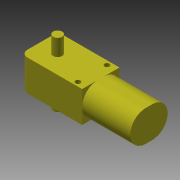
# Autodesk Inventor part: Motor_gerade
Saved by Autodesk Inventor 2015 (Build 190159000, 159)
## iProperties
Created: 2015-03-02
Part Number: Motor_gerade
Material: Generisch
Document SubType Name: Modeling
Designer: TowerSebi
Density: 1 g/cm^3
Appearance: Kanariengelb
Author: TowerSebi
Autodesk Inventor part; units mm, degrees
ref_plane "YZ Plane" through (0, 0, 0) normal (1, 0, 0) x (0, 1, 0)
ref_plane "XZ Plane" through (0, 0, 0) normal (0, 1, 0) x (-1, 0, 0)
ref_plane "XY Plane" through (0, 0, 0) normal (0, 0, 1) x (1, 0, 0)
sketch "Skizze1" plane through (0, 0, 0) normal (0, 0, 1) x (1, 0, 0)
  line L0 (0, 0) -> (37, 0)
  line L1 (37, 0) -> (37, 22.5)
  line L2 (37, 22.5) -> (0, 22.5)
  line L3 (0, 22.5) -> (0, 0)
  dimension "d0" = 37
  dimension "d1" = 22.5
  constraints: 8 end point, 2 parallel, 1 horizontal, 1 perpendicular
  measures "d0" distance of L1.end L2.end
  measures "d1" distance of L2.end L0.start
extrude "Extrusion1" add sketch "Skizze1" along normal blind 18.7
sketch "Skizze2" plane through (37, 0, 0) normal (1, 0, 0) x (0, 0, -1)
  line L0 (0, 0) -> (0, 22.5) projected
  line L1 (-9.35, 13.157) -> (-9.35, 9.3514) construction
  line L2 (-18.7, 13.157) -> (-18.7, 9.3514)
  line L3 (0, 9.3514) -> (0, 13.157)
  arc A0 (0, 13.157) -> (-18.7, 13.157) centre (-9.35, 13.157) ccw
  arc A1 (-18.7, 9.3514) -> (0, 9.3514) centre (-9.35, 9.3514) ccw
  point P0 (-9.35, 11.2542)
  constraints: 8 end point, 4 point on circle, 4 tangent, 2 centre point, 2 parallel, 1 midpoint
extrude "Extrusion2" add sketch "Skizze2" along normal blind 29
sketch "Skizze3" plane through (0, 0, 18.7) normal (0, 0, 1) x (1, 0, 0)
  line L0 (37, 22.5) -> (0, 22.5) projected
  line L1 (0, 22.5) -> (0, 0) projected
  circle A0 centre (11, 11.25) radius 2.75
  dimension "d6" = 11
  dimension "d7" = 11.25
  dimension "d21" = 5.5
  constraints: 1 centre point
  measures "d6" distance from line of L1 A0.centre
  measures "d7" distance from line of L0 A0.centre
  measures "d21" diameter of A0
extrude "Extrusion3" add sketch "Skizze3" along normal blind 10
sketch "Skizze4" plane through (0, 0, 0) normal (0, 0, -1) x (-1, 0, 0)
  line L0 (0, 0) -> (-37, 0) projected
  line L1 (0, 22.5) -> (0, 0) projected
  circle A0 centre (-11, 11.25) radius 2.75
  dimension "d10" = 5.5
  dimension "d11" = 11
  dimension "d12" = 11.25
  constraints: 1 centre point
  measures "d10" diameter of A0
  measures "d11" distance from line of L1 A0.centre
  measures "d12" distance from line of L0 A0.centre
extrude "Extrusion4" add sketch "Skizze4" along normal blind 10
sketch "Skizze5" plane through (0, 0, 0) normal (0, 0, -1) x (-1, 0, 0)
  line L0 (0, 0) -> (-37, 0) projected
  line L1 (0, 22.5) -> (0, 0) projected
  line L2 (-37, 22.5) -> (0, 22.5) projected
  circle A0 centre (-22.5, 11.25) radius 2
  dimension "d15" = 4
  dimension "d16" = 11.25
  dimension "d17" = 22.5
  dimension "d18" = 11.25
  constraints: 1 centre point
  measures "d15" diameter of A0
  measures "d16" distance from line of L0 A0.centre
  measures "d17" distance from line of L1 A0.centre
  measures "d18" distance from line of L2 A0.centre
extrude "Extrusion5" add sketch "Skizze5" along normal blind 2
sketch "Skizze6" plane through (0, 0, 0) normal (-1, 0, 0) x (0, 0, 1)
  line L0 (0, 22.5) -> (0, 0) projected
  line L1 (18.7, 22.5) -> (18.7, 0) projected
  line L2 (7.85, 13.5868) -> (10.85, 13.5868)
  line L3 (10.85, 13.5868) -> (10.85, 8.5868)
  line L4 (10.85, 8.5868) -> (7.85, 8.5868)
  line L5 (7.85, 8.5868) -> (7.85, 13.5868)
  line L6 (9.35, 13.5868) -> (9.35, 8.5868)
  dimension "d22" = 3
  dimension "d23" = 5
  dimension "d25" = 18.7
  dimension "d26" = 7.85
  dimension "d27" = 7.85
  constraints: 10 end point, 2 midpoint, 2 parallel, 1 horizontal, 1 perpendicular
  measures "d22" distance of L2.start L2.end
  measures "d23" distance of L2.end L3.end
  measures "d25" distance between parallel lines of L1 L0
  measures "d26" distance between parallel lines of L0 L5
  measures "d27" distance between parallel lines of L1 L3
extrude "Extrusion6" add sketch "Skizze6" along normal blind 5
fillet "Rundung1" radius 4 2 edges at (0, 22.5, 9.35) (0, 0, 9.35)
sketch "Skizze7" plane through (0, 0, 18.7) normal (0, 0, 1) x (1, 0, 0)
  line L0 (4, 0) -> (37, 0) projected
  line L1 (37, 22.5) -> (4, 22.5) projected
  line L2 (0, 18.5) -> (0, 4) projected
  circle A0 centre (32, 20) radius 1.5
  circle A1 centre (32, 2.5) radius 1.5
  point P0 (0, 0)
  dimension "d31" = 2.5
  dimension "d32" = 2.5
  dimension "d33" = 32
  dimension "d34" = 32
  dimension "d35" = 3
  dimension "d36" = 3
  constraints: 2 centre point
  measures "d31" distance from line of L1 A0.centre
  measures "d32" distance from line of L0 A1.centre
  measures "d33" distance from line of A1.centre L2
  measures "d34" distance from line of L2 A0.centre
  measures "d35" diameter of A0
  measures "d36" diameter of A1
extrude "Extrusion7" cut sketch "Skizze7" against normal up to next
hole "Bohrung1" at (-2.5, 11.0868, 10.85) direction (0, 0, -1) diameter 3 end through all
